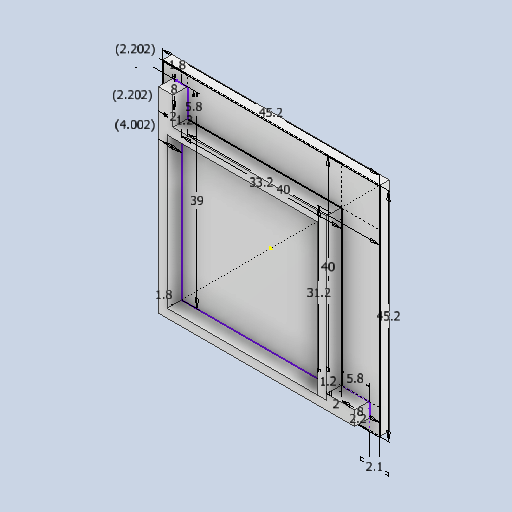
# Autodesk Inventor part: DownCover
Saved by Autodesk Inventor 2023 (Build 270158000, 158)
## iProperties
Created: 2022-08-19
Part Number: DownCover
Material: ABS Plastic
Document SubType Name: Modeling
Designer: Miner
Density: 1.06 g/cm^3
Appearance: Smooth - White
Author: Miner
Autodesk Inventor part; units mm, degrees
ref_plane "YZ Plane" through (0, 0, 0) normal (1, 0, 0) x (0, 1, 0)
ref_plane "XZ Plane" through (0, 0, 0) normal (0, 1, 0) x (-1, 0, 0)
ref_plane "XY Plane" through (0, 0, 0) normal (0, 0, 1) x (1, 0, 0)
sketch "Sketch1" plane through (0, 0, 0) normal (0, 0, 1) x (1, 0, 0)
  line L0 (-22.6, -22.6) -> (22.6, -22.6)
  line L1 (22.6, -22.6) -> (22.6, 22.6)
  line L2 (22.6, 22.6) -> (-22.6, 22.6)
  line L3 (-22.6, 22.6) -> (-22.6, -22.6)
  line L4 (-22.6, -22.6) -> (22.6, 22.6) construction
  line L5 (22.6, -22.6) -> (20.5, -22.6) construction
  line L6 (20.5, -22.6) -> (20.4022, -20.4022) construction
  line L7 (20.4022, -20.4022) -> (-20.3978, -20.4022)
  line L8 (-20.3978, -20.4022) -> (-20.3978, -18.6022)
  line L9 (-20.3978, -18.6022) -> (20.4022, -18.6022)
  line L10 (20.4022, -18.6022) -> (20.4022, -20.4022)
  line L11 (-20.3978, -18.6022) -> (-18.5978, -18.6022)
  line L12 (-18.5978, -18.6022) -> (-18.5978, 20.3978)
  line L13 (-18.5978, 20.3978) -> (-20.3978, 20.3978)
  line L14 (-20.3978, 20.3978) -> (-20.3978, -18.6022)
  line L15 (-18.5978, 20.3978) -> (-17.3978, 20.3978)
  line L16 (-17.3978, 20.3978) -> (-17.3978, 14.5978)
  line L17 (-17.3978, 14.5978) -> (-18.5978, 14.5978)
  line L18 (-18.5978, 14.5978) -> (-18.5978, 20.3978)
  line L19 (20.4022, -18.6022) -> (14.6022, -18.6022)
  line L20 (14.6022, -18.6022) -> (14.6022, -17.4022)
  line L21 (14.6022, -17.4022) -> (20.4022, -17.4022)
  line L22 (20.4022, -17.4022) -> (20.4022, -18.6022)
  line L23 (22.6, 22.6) -> (-17.4, 22.6) construction
  line L24 (-17.4, 22.6) -> (-17.4, 14.6) construction
  line L25 (-17.4, 14.6) -> (22.6, 14.6) construction
  line L26 (22.6, 14.6) -> (22.6, 22.6) construction
  line L27 (22.6, 22.6) -> (14.6, 22.6) construction
  line L28 (14.6, 22.6) -> (14.6, -17.4) construction
  line L29 (14.6, -17.4) -> (22.6, -17.4) construction
  line L30 (22.6, -17.4) -> (22.6, 22.6) construction
  line L31 (14.6, 14.6) -> (-18.6, 14.6)
  line L32 (-18.6, 14.6) -> (-18.6, 12.6)
  line L33 (-18.6, 12.6) -> (14.6, 12.6)
  line L34 (14.6, 12.6) -> (14.6, 14.6)
  line L35 (14.6, 12.6) -> (12.6, 12.6)
  line L36 (12.6, 12.6) -> (12.6, -18.6)
  line L37 (12.6, -18.6) -> (14.6, -18.6)
  line L38 (14.6, -18.6) -> (14.6, 12.6)
  point P0 (0, 0)
  point P1 (-19.4978, 20.3978)
  point P2 (-17.3978, 14.6)
  point P3 (-18.5978, 12.6)
  dimension "d0" = 45.2
  dimension "d1" = 45.2
  dimension "d2" = 2.1
  dimension "d3" = 2.2
  dimension "d5" = 1.8
  dimension "d6" = 1.8
  dimension "d7" = 39
  dimension "d10" = 2.2022
  dimension "d11" = 4.0022
  dimension "d12" = 2.2022
  dimension "d15" = 1.2
  dimension "d16" = 5.8
  dimension "d21" = 5.8
  dimension "d22" = 1.2
  dimension "d25" = 40
  dimension "d26" = 8
  dimension "d27" = 8
  dimension "d28" = 40
  dimension "d29" = 33.2
  dimension "d30" = 2
  dimension "d31" = 2
  dimension "d32" = 31.2
  constraints: 78 end point, 18 parallel, 9 horizontal, 9 perpendicular, 3 point on line, 2 midpoint
  measures "d0" distance of L2.end L1.end
  measures "d1" distance of L1.end L0.end
  measures "d2" distance of L0.end L5.end
  measures "d3" distance of L5.end L6.end
  measures "d5" distance of L7.end L8.end
  measures "d6" distance of L13.end L12.end
  measures "d7" distance of L12.end L11.end
  measures "d10" distance between parallel lines of L3 L14
  measures "d11" distance between parallel lines of L12 L3
  measures "d12" distance from line of point (-19.498, 20.398) L2
  measures "d15" distance of L16.end L17.end
  measures "d16" distance of L15.end L16.end
  measures "d21" distance of L20.end L21.end
  measures "d22" distance of L19.end L20.end
  measures "d25" distance of L25.end L24.end
  measures "d26" distance of L24.end L23.end
  measures "d27" distance of L29.end L28.end
  measures "d28" distance of L28.end L27.end
  measures "d29" distance of L33.end L32.end
  measures "d30" distance of L32.end L31.end
  measures "d31" distance of L37.end L36.end
  measures "d32" distance of L36.end L35.end
extrude "Extrusion1" add sketch "Sketch1" along normal blind 3 contours L7 L8 L9 L10 | L14 L13 L12 L31 L32 L33 L9 | L33 L32 L31 L12
extrude "Extrusion2" add sketch "Sketch1" against normal blind 2 contours L3 L2 L1 L0 | L7 L8 L9 L10 | L9 L20 L21 L22 | L14 L13 L12 L31 L32 L33 L9 | L33 L32 L31 L12 | L12 L17 L16 L31 L34 L33 | L15 L16 L31 L12 | L12 L31 L16 L17 | L33 L38 L37 L36
extrude "Extrusion4" add sketch "Sketch1" along normal blind 3 contours L9 L20 L21 L22 | L15 L16 L31 L12 | L12 L31 L16 L17
extrude "Extrusion5" add sketch "Sketch1" along normal blind 3 contours L12 L17 L16 L31 L34 L33 | L33 L38 L37 L36
fillet "Fillet1" radius 1 1 edges at (-22.6, -22.6, -1)
body "Solid1"
